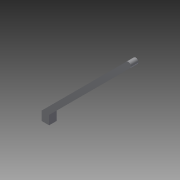
# Autodesk Inventor part: Funneling_v1
Saved by Autodesk Inventor 2013 (Build 170138000, 138)
## iProperties
Created: 2013-01-19
Part Number: Funneling_v1
Material: Generic
Document SubType Name: Modeling
Designer: motoennies
Density: 1 g/cm^3
Mass: 3.19039 g
Surface Area: 24.4853 cm^2
Volume: 3.19039 cm^3
Author: motoennies
Autodesk Inventor part; units mm, degrees
ref_plane "YZ Plane" through (0, 0, 0) normal (1, 0, 0) x (0, 1, 0)
ref_plane "XZ Plane" through (0, 0, 0) normal (0, 1, 0) x (-1, 0, 0)
ref_plane "XY Plane" through (0, 0, 0) normal (0, 0, 1) x (1, 0, 0)
sketch "Sketch1" plane through (0, 0, 0) normal (0, 0, 1) x (1, 0, 0)
  line L0 (0, 0) -> (0, 7.62)
  line L1 (0, 0) -> (6.35, 0)
  line L2 (0, 7.62) -> (73.3235, 7.62) construction
  line L3 (6.35, 0) -> (6.35, 7.62)
  line L4 (6.35, 7.62) -> (13.3564, 7.62) construction
  line L5 (0, 7.62) -> (71.842, 79.462)
  line L6 (6.35, 7.62) -> (75.017, 76.287)
  arc A0 (75.017, 76.287) -> (71.842, 79.462) centre (73.4295, 77.8745) ccw
  dimension "d0" = 7.62
  dimension "d1" = 6.35
  dimension "d8" = 7.62
  dimension "d27" = 101.6
  dimension "d28" = 45
  constraints: 14 end point, 2 horizontal, 2 point on circle, 1 centre point, 1 parallel, 1 perpendicular, 1 point on line, 1 vertical
  measures "d0" distance of L0.start L0.end
  measures "d1" distance of L0.start L1.end
  measures "d8" distance of L1.end L3.end
  measures "d27" distance of L0.end L5.end
  measures "d28" angle of L2 L5
extrude "Extrusion4" add sketch "Sketch1" along normal blind 6.35
body "Solid4"
